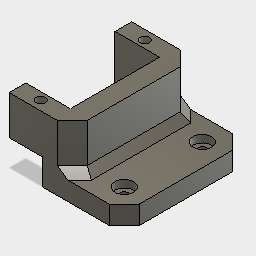
bar-latch-servo-shim (Autodesk Fusion 360 design; units mm, degrees)
Autodesk Fusion 360 part; units mm, degrees
box "BoxPrimitive1" add length 33 width 31 height 5 placed x (0, 0, 1) y (1, 0, 0) z (0, 1, 0) at (0, 0, 0) makes body 1
box "BoxPrimitive2" add length 33 width 17 height 12.5 placed x (0, 0, 1) y (1, 0, 0) z (0, 1, 0) at (0, 5, 0) bodies 1
box "BoxPrimitive3" add length 24 width 25 height 30 placed x (0, 0, 1) y (1, 0, 0) z (0, 1, 0) at (-30, 0, 0) separate body makes body 2
move_body "MoveBody1" bodies 2 to x (1, 0, 0) y (0, 1, 0) z (0, 0, 1) at (5, 0, 4.5)
move_body "MoveBody2" bodies 2 to x (1, 0, 0) y (0, 1, 0) z (0, 0, 1) at (12, 0, 0)
combine "Combine1" operation cut target body 1 tool bodies 2
hole "Hole1" at (6, 17.5, 2.5) direction (0, -1, 0) diameter 2.5 depth 8 tip angle 118 bodies 1
hole "Hole2" at (6, 17.5, 30.5) direction (0, -1, 0) diameter 2.5 depth 8 tip angle 118 bodies 1
hole "Hole3" at (25, 5, 6) direction (0, -1, 0) diameter 2.5 depth 8 tip angle 118 counterbore diameter 5 counterbore depth 2 bodies 1
hole "Hole4" at (25, 5, 27) direction (0, -1, 0) diameter 2.5 depth 8 tip angle 118 counterbore diameter 5 counterbore depth 2 bodies 1
box "BoxPrimitive4" cut length 7 width 9 height -12 placed x (0, 1, 0) y (-1, 0, 0) z (0, 0, 1) at (9, 0, 33) bodies 1
chamfer "Chamfer1" distance 4 angle 45 4 edges at (17, 11.25, 33) (17, 11.25, 0) (31, 2.5, 33) (31, 2.5, 0) on bodies 1
chamfer "Chamfer2" distance 2 angle 45 3 edges at (17, 5, 16.5) (15, 5, 31) (15, 5, 2) on bodies 1
